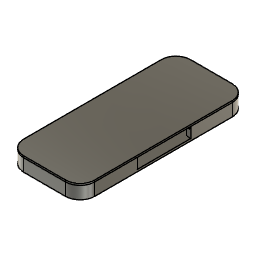
case with offset lid_ (Autodesk Fusion 360 design; units mm, degrees)
Autodesk Fusion 360 part; units mm, degrees
sketch "Sketch1" plane through (0, 0, 0) normal (0, 0, 1) x (1, 0, 0)
  circle A0 centre (6.1655, 9.1526) radius 11.625
  dimension "d1" = 23.25
  measures "d1" diameter of A0
sketch "Sketch2" plane through (0, 0, 0) normal (0, 0, 1) x (1, 0, 0)
  line L0 (-57.9255, -30.9161) -> (-77.9255, -30.9161)
  line L1 (-82.9255, -25.9161) -> (-82.9255, 40)
  line L2 (-77.9255, 45) -> (-57.9255, 45)
  line L3 (-52.9255, 40) -> (-52.9255, -25.9161)
  arc A0 (-77.9255, 45) -> (-82.9255, 40) centre (-77.9255, 40) ccw
  arc A1 (-52.9255, 40) -> (-57.9255, 45) centre (-57.9255, 40) ccw
  arc A2 (-82.9255, -25.9161) -> (-77.9255, -30.9161) centre (-77.9255, -25.9161) ccw
  arc A3 (-57.9255, -30.9161) -> (-52.9255, -25.9161) centre (-57.9255, -25.9161) ccw
  arc A4 (-77.9255, 47) -> (-84.9255, 40) centre (-77.9255, 40) ccw
  line L4 (-84.9255, -25.9161) -> (-84.9255, 40)
  arc A5 (-84.9255, -25.9161) -> (-77.9255, -32.9161) centre (-77.9255, -25.9161) ccw
  line L5 (-57.9255, -32.9161) -> (-77.9255, -32.9161)
  arc A6 (-57.9255, -32.9161) -> (-50.9255, -25.9161) centre (-57.9255, -25.9161) ccw
  line L6 (-50.9255, 40) -> (-50.9255, -25.9161)
  arc A7 (-50.9255, 40) -> (-57.9255, 47) centre (-57.9255, 40) ccw
  line L7 (-77.9255, 47) -> (-57.9255, 47)
  dimension "d2" = 5
  dimension "d3" = 5
  dimension "d4" = 5
  dimension "d5" = -2
  dimension "d17" = 30
  constraint horizontal L0
  constraint vertical L1
  constraint horizontal L2
  constraint vertical L3
  constraint tangent L1 A0
  constraint tangent L2 A0
  constraint tangent L2 A1
  constraint tangent L3 A1
  constraint tangent L0 A2
  constraint tangent L1 A2
  constraint equal A1 A2
  constraint tangent L0 A3
  constraint tangent L3 A3
  measures "d2" radius of A0
  measures "d3" radius of A1
  measures "d4" radius of A3
  measures "d17" distance of L1 L3
extrude "Extrude2" add sketch "Sketch2" along normal blind 1 contours L0 L1 L2 L3 A0 A1 A2 A3 makes body 1
extrude "Extrude3" add sketch "Sketch2" along normal blind 6 bodies 1
sketch "Sketch3" plane through (0, 0, 0) normal (0, 0, 1) x (1, 0, 0)
sketch "Sketch4" plane through (-50.9255, 0, 0) normal (1, 0, 0) x (0, 1, 0)
  line L0 (-25.9161, 0) -> (40, 0)
  line L1 (40, 0) -> (40, 6)
  line L2 (40, 6) -> (-25.9161, 6)
  line L3 (-25.9161, 6) -> (-25.9161, 0)
  line L4 (-5.5081, 6) -> (20.1819, 6)
  line L5 (20.1819, 6) -> (20.1819, 1)
  line L6 (20.1819, 1) -> (-5.5081, 1)
  line L7 (-5.5081, 1) -> (-5.5081, 6)
  dimension "d12" = 25.69
  dimension "d13" = 5
  dimension "d14" = 20.408
  constraint horizontal L4
  constraint vertical L5
  constraint horizontal L6
  constraint vertical L7
  constraint coincident L2 L4.start
  measures "d12" distance of L4.start L4.end
  measures "d13" distance of L4.start L6.end
  measures "d14" distance of L3 L7
extrude "Extrude4" cut sketch "Sketch4" against normal blind 2 contours L2 L4 L5 L6 L7 bodies 1
ref_plane "WorkPlane1" through (-67.9255, 7.0419, 6) normal (0, 0, 1) x (1, 0, 0)
sketch "Sketch14" plane through (0, 0, 6) normal (0, 0, 1) x (1, 0, 0)
  line L0 (-84.9255, -25.9161) -> (-84.9255, 40)
  arc A0 (-77.9255, 47) -> (-84.9255, 40) centre (-77.9255, 40) ccw
  line L1 (-77.9255, 47) -> (-57.9255, 47)
  arc A1 (-50.9255, 40) -> (-57.9255, 47) centre (-57.9255, 40) ccw
  line L2 (-50.9255, 40) -> (-50.9255, -25.9161)
  arc A2 (-57.9255, -32.9161) -> (-50.9255, -25.9161) centre (-57.9255, -25.9161) ccw
  line L3 (-57.9255, -32.9161) -> (-77.9255, -32.9161)
  arc A3 (-84.9255, -25.9161) -> (-77.9255, -32.9161) centre (-77.9255, -25.9161) ccw
extrude "Extrude5" add sketch "Sketch14" along normal blind 0.8 separate body makes body 2
sketch "Sketch15" plane through (0, 0, 6) normal (0, 0, 1) x (1, 0, 0)
  arc A0 (-82.9255, -25.9161) -> (-77.9255, -30.9161) centre (-77.9255, -25.9161) ccw
  line L0 (-77.9255, -30.9161) -> (-57.9255, -30.9161)
  arc A1 (-57.9255, -30.9161) -> (-52.9255, -25.9161) centre (-57.9255, -25.9161) ccw
  line L1 (-52.9255, -25.9161) -> (-52.9255, -5.5081)
  line L2 (-52.9255, -5.5081) -> (-50.9255, -5.5081)
  line L3 (-50.9255, -5.5081) -> (-50.9255, 20.1819)
  line L4 (-50.9255, 20.1819) -> (-52.9255, 20.1819)
  line L5 (-52.9255, 20.1819) -> (-52.9255, 40)
  arc A2 (-52.9255, 40) -> (-57.9255, 45) centre (-57.9255, 40) ccw
  line L6 (-57.9255, 45) -> (-77.9255, 45)
  arc A3 (-77.9255, 45) -> (-82.9255, 40) centre (-77.9255, 40) ccw
  line L7 (-82.9255, 40) -> (-82.9255, -25.9161)
  line L8 (-51.1255, -5.3081) -> (-51.1255, 19.9819)
  line L9 (-51.1255, 19.9819) -> (-53.1255, 19.9819)
  line L10 (-53.1255, 19.9819) -> (-53.1255, 40)
  arc A4 (-53.1255, 40) -> (-57.9255, 44.8) centre (-57.9255, 40) ccw
  line L11 (-57.9255, 44.8) -> (-77.9255, 44.8)
  arc A5 (-77.9255, 44.8) -> (-82.7255, 40) centre (-77.9255, 40) ccw
  line L12 (-82.7255, 40) -> (-82.7255, -25.9161)
  arc A6 (-82.7255, -25.9161) -> (-77.9255, -30.7161) centre (-77.9255, -25.9161) ccw
  line L13 (-77.9255, -30.7161) -> (-57.9255, -30.7161)
  arc A7 (-57.9255, -30.7161) -> (-53.1255, -25.9161) centre (-57.9255, -25.9161) ccw
  line L14 (-53.1255, -25.9161) -> (-53.1255, -5.3081)
  line L15 (-53.1255, -5.3081) -> (-51.1255, -5.3081)
  dimension "d25" = -0.2
extrude "Extrude8" add sketch "Sketch15" against normal blind 1.2 contours L8 L9 L10 A4 L11 A5 L12 A6 L13 A7 L14 L15 bodies 2
sketch "Sketch17" plane through (0, 0, 4.8) normal (0, 0, -1) x (1, 0, 0)
  line L0 (-51.1255, 5.3081) -> (-53.1255, 5.3081)
  line L1 (-53.1255, 5.3081) -> (-53.1255, 25.9161)
  arc A0 (-53.1255, 25.9161) -> (-57.9255, 30.7161) centre (-57.9255, 25.9161) ccw
  line L2 (-57.9255, 30.7161) -> (-77.9255, 30.7161)
  arc A1 (-77.9255, 30.7161) -> (-82.7255, 25.9161) centre (-77.9255, 25.9161) ccw
  line L3 (-82.7255, 25.9161) -> (-82.7255, -40)
  arc A2 (-82.7255, -40) -> (-77.9255, -44.8) centre (-77.9255, -40) ccw
  line L4 (-77.9255, -44.8) -> (-57.9255, -44.8)
  arc A3 (-57.9255, -44.8) -> (-53.1255, -40) centre (-57.9255, -40) ccw
  line L5 (-53.1255, -40) -> (-53.1255, -19.9819)
  line L6 (-53.1255, -19.9819) -> (-51.1255, -19.9819)
  line L7 (-51.1255, -19.9819) -> (-51.1255, 5.3081)
  circle A4 centre (-51.1255, -7.3369) radius 12.645
  constraint coincident L6.end A4
  constraint tangent L6 A4
  constraint coincident L0.start A4
extrude "Extrude9" cut sketch "Sketch17" against normal blind 1.2 contours L7 A4 picked at (-52.9961, -11.4117) bodies 2
